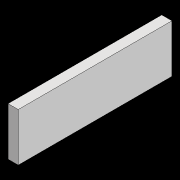
# Autodesk Inventor part: 垂直アーム(仮)
Saved by Autodesk Inventor 2022 (Build 260153000, 153)
## iProperties
Created: 2021-07-07
Part Number: 垂直アーム(仮)
Material: 一般
Document SubType Name: Modeling
Designer: nrz71
Density: 1 g/cm^3
Appearance: 既定
Author: nrz71
Autodesk Inventor part; units mm, degrees
ref_plane "YZ Plane" through (0, 0, 0) normal (1, 0, 0) x (0, 1, 0)
ref_plane "XZ Plane" through (0, 0, 0) normal (0, 1, 0) x (-1, 0, 0)
ref_plane "XY Plane" through (0, 0, 0) normal (0, 0, 1) x (1, 0, 0)
sketch "スケッチ1" plane through (0, 0, 0) normal (1, 0, 0) x (0, 1, 0)
  line L0 (0, 0) -> (-66, 0)
  line L1 (-66, 0) -> (-66, 302.0596)
  line L2 (-66, 302.0596) -> (0, 302.0596)
  line L3 (0, 302.0596) -> (0, 0)
  dimension "d9" = 66
  constraints: 8 end point, 2 parallel, 1 horizontal, 1 perpendicular
  measures "d9" distance of L0.start L0.end
extrude "押し出し1" add sketch "スケッチ1" along normal blind 20
sketch "スケッチ2" plane through (0, -66, 0) normal (0, -1, 0) x (1, 0, 0)
  point P0 (0, 0)
  point P1 (10.6073, 293.7876)
hole "穴1" at (10.6073, -66, 293.7876) direction (0, 1, 0) diameter 10 end through all
